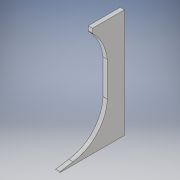
# Autodesk Inventor part: New Shooter Curve
Saved by Autodesk Inventor 2018 (Build 220112000, 112)
## iProperties
Created: 2020-02-18
Part Number: New Shooter Curve
Material: Generic
Document SubType Name: Modeling
Designer: T3500STATIC
Density: 1 g/cm^3
Appearance: Default
Author: T3500STATIC
Autodesk Inventor part; units mm, degrees
ref_plane "YZ Plane" through (0, 0, 0) normal (1, 0, 0) x (0, 1, 0)
ref_plane "XZ Plane" through (0, 0, 0) normal (0, 1, 0) x (-1, 0, 0)
ref_plane "XY Plane" through (0, 0, 0) normal (0, 0, 1) x (1, 0, 0)
sketch "Sketch1" plane through (0, 0, 0) normal (1, 0, 0) x (0, 1, 0)
  line L0 (0, 0) -> (330.2, 0) construction
  line L1 (330.2, 0) -> (330.2, 304.8)
  line L2 (330.2, 304.8) -> (0, 304.8) construction
  line L3 (0, 304.8) -> (0, 0)
  line L4 (0, 0) -> (482.6, 0)
  line L5 (482.6, 0) -> (482.6, 76.2) construction
  line L6 (482.6, 76.2) -> (0, 76.2)
  line L7 (0, 76.2) -> (0, 0) construction
  circle A0 centre (330.2, 304.8) radius 76.2
  line L8 (330.2, 304.8) -> (462.0741, 141.9491) construction
  line L9 (330.2, 304.8) -> (330.2, 76.2) construction
  line L10 (330.2, 304.8) -> (403.3287, 98.2908) construction
  arc A1 (330.2, 76.2) -> (462.0741, 141.9491) centre (304.8762, 292.1181) ccw
  line L11 (330.2, 304.8) -> (254, 304.8) construction
  line L12 (254, 304.8) -> (254, 228.6) construction
  line L13 (254, 228.6) -> (330.2, 228.6) construction
  line L14 (330.2, 228.6) -> (330.2, 304.8) construction
  line L15 (254, 228.6) -> (441.325, 228.6) construction
  circle A2 centre (254, 228.6) radius 6.35
  line L16 (254, 228.6) -> (241.3, 76.2) construction
  line L17 (254, 228.6) -> (419.1, 228.6) construction
  line L18 (0, 76.2) -> (190.5, 76.2) construction
  line L19 (190.5, 76.2) -> (190.5, 228.6) construction
  line L20 (190.5, 228.6) -> (0, 228.6) construction
  line L21 (0, 228.6) -> (0, 76.2) construction
  circle A3 centre (190.5, 228.6) radius 6.35
  line L22 (190.5, 228.6) -> (76.0017, 114.1017) construction
  line L23 (190.5, 228.6) -> (352.425, 228.6) construction
  line L24 (190.5, 228.6) -> (12.7, 228.6) construction
  arc A4 (12.7, 228.6) -> (190.5, 76.2) centre (184.0395, 248.5794) ccw
  line L25 (12.7, 228.6) -> (0, 304.8)
  line L26 (462.0741, 141.9491) -> (482.6, 141.9491)
  line L27 (482.6, 141.9491) -> (482.6, 0)
  line L28 (330.2, 76.2) -> (177.5789, 76.2)
  dimension "d0" = 330.2
  dimension "d1" = 304.8
  dimension "d2" = 482.6
  dimension "d3" = 76.2
  dimension "d4" = 152.4
  dimension "d5" = 209.55
  dimension "d9" = 228.6
  dimension "d13" = 219.075
  dimension "d16" = 39
  dimension "d17" = 19.5
  dimension "d19" = 76.2
  dimension "d20" = 76.2
  dimension "d25" = 12.7
  dimension "d39" = 190.5
  dimension "d40" = 152.4
  dimension "d41" = 12.7
  dimension "d42" = 161.925
  dimension "d43" = 135
  dimension "d44" = 177.8
  constraints: 58 end point, 8 horizontal, 8 parallel, 7 point on circle, 5 centre point, 4 coincident, 4 perpendicular, 3 point on line, 1 collinear, 1 equal length, 1 midpoint
  measures "d0" distance of L2.end L1.end
  measures "d1" distance of L1.end L0.end
  measures "d2" distance of L6.end L5.end
  measures "d3" distance of L5.end L4.end
  measures "d4" diameter of A0
  measures "d5" distance of L8.start L8.end
  measures "d9" distance of L8.start L9.end
  measures "d13" distance of L8.start L10.end
  measures "d16" angle of L1 L8
  measures "d17" angle of L1 L10
  measures "d19" distance of L13.end L12.end
  measures "d20" distance of L12.end L11.end
  measures "d25" diameter of A2
  measures "d39" distance of L20.end L19.end
  measures "d40" distance of L19.end L18.end
  measures "d41" diameter of A3
  measures "d42" distance of L22.start L22.end
  measures "d43" angle of L22 L23
  measures "d44" distance of L22.start L24.end
extrude "Extrusion1" add sketch "Sketch1" along normal blind 19.05 contours L4 L3 L6 A4 L1 | L1 L6 L27 L4 | A1 L26 L27 L6 | A4 L6 | L3 L25 A4 L6
fillet "Fillet1" radius 1.5875 1 edges at (9.525, 0, 304.8)
fillet "Fillet2" radius 3.175 1 edges at (9.525, 462.0741, 141.9491)
body "Solid1"
